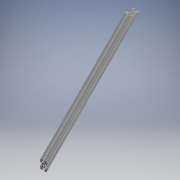
# Autodesk Inventor part: HFBL5-2020-300_
Saved by Autodesk Inventor 2017.3 (Build 213256000, 256)
## iProperties
Part Number: HFBL5-2020-300_
Material: Generic
Catalog Web Link: www.cadenas.de
Description: HFBL5_-Brackets HFS5 Frame Brackets for Reinforcement
Vendor: MISUMI
Document SubType Name: Modeling
Designer: partserver
Manufacturer: MISUMI
Mass: 73.1525 g
Surface Area: 703.124 cm^2
Volume: 73.1525 cm^3
Density: 1 g/cm^3
Appearance: PSOLRGB-192-192-192
Category: PARTsolutions
Company: MISUMI
Title: HFBL5-2020-300_
Author: Cadenas PARTsolutions
Comments: Brackets HFS5 Frame Brackets for Reinforcement
PSOL_IDENT_0: {$CADENAS_DATA\23d-libs\misumi\metric\38_al_extrusions_blackets\5\hfbl5.prj},176 {VTYP=3D},{NB=HFBL5
PSOL_IDENT_1: -2020-300_},{LINA=HFBL5-2020-300_},{NN=HFBL5_},{DATE=08.06.2021 08:25:15},{GEOMDATE=30.01.2015 00:00
PSOL_IDENT_2: :00},{VERSION=},{LINEID=10},{WBVAR=L,ALT},{WBNUMERIC=L}  {NB=HFBL5-2020-300_},{LINA=HFBL5-2020-300_}
PSOL_IDENT_3: ,{KT=1},{PN=HFBL5-2020-300},{TP=HFBL5},{NO=2020},{TYPE=HFBL5},{MAT=A6N01SS-T5},{ST=Alumite Treatment
PSOL_IDENT_4: (No surface treatment on the side cut at 45 degree and  Counterbore type)},{FEAT=4 Slots},{L=300},{
PSOL_IDENT_5: LTOL=+/- 0.5},{MASS=0.50},{SA=153},{GMILX=0.57x10^4},{GMILY=0.57x10^4},{WIDTH=20},{HEIGHT=20},{TAPDE
PSOL_IDENT_6: PTH=15},{TAPSTART=0},{DRILLLENGTH=0},{DRILLDIA=4.2},{TAPPOSHOR=0},{TAPPOSVER=0},{VER=1},{DIM=1},{CLF=
PSOL_IDENT_7: HFS5-2020},{ALT3=},{AB=CBM5-8},{ABQ=2},{AN=HNTT5-5},{ANQ=2},{ALT=}
NB: HFBL5-2020-300_
NN: HFBL5_
NT: Brackets HFS5 Frame Brackets for Reinforcement
NBSYN: $PN._
LINA: HFBL5-2020-300_
CATALOG: Misumi
PN: HFBL5-2020-300
NO: 2020
MAT: A6N01SS-T5 Aluminum Alloy
ST: Alumite Treatment (No surface treatment on the side cut at 45 degree and  Counterbore type)
L: 300
WIDTH: 20
AB: CBM5-8
ABQ: 2
AN: HNTT5-5
ANQ: 2
ALT: w/o Set of Applicable Bolt and Nut
SUPPLIER: MISUMI
ARTICLENO: HFBL5-2020-300_
BOMINFO: HFBL5-2020-300_
CREATOR: CADENAS GmbH
Autodesk Inventor part; units mm, degrees
sketch "Sketch_1" plane through (0, 0, 0) normal (0, -0.7071068, 0.7071068) x (1, 0, 0)
  arc A0 (-10, 205.432) -> (-9.7, 205.132) centre (-9.7, 205.432) ccw
  line L0 (-9.7, 205.132) -> (-8, 205.132)
  line L1 (-8, 205.132) -> (-8, 208.132)
  line L2 (-8, 208.132) -> (-7.0607, 208.132)
  line L3 (-7.0607, 208.132) -> (-4, 205.0714)
  line L4 (-4, 205.0714) -> (-4, 202.432)
  line L5 (-4, 202.432) -> (-3.7, 202.132)
  line L6 (-3.7, 202.132) -> (-4, 201.832)
  line L7 (-4, 201.832) -> (-4, 199.1927)
  line L8 (-4, 199.1927) -> (-7.0607, 196.132)
  line L9 (-7.0607, 196.132) -> (-8, 196.132)
  line L10 (-8, 196.132) -> (-8, 199.132)
  line L11 (-8, 199.132) -> (-9.7, 199.132)
  arc A1 (-9.7, 199.132) -> (-10, 198.832) centre (-9.7, 198.832) ccw
  line L12 (-10, 198.832) -> (-10, 193.132)
  arc A2 (-10, 193.132) -> (-9, 192.132) centre (-9, 193.132) ccw
  line L13 (-9, 192.132) -> (-3.3, 192.132)
  arc A3 (-3.3, 192.132) -> (-3, 192.432) centre (-3.3, 192.432) ccw
  line L14 (-3, 192.432) -> (-3, 194.132)
  line L15 (-3, 194.132) -> (-6, 194.132)
  line L16 (-6, 194.132) -> (-6, 195.0714)
  line L17 (-6, 195.0714) -> (-2.9393, 198.132)
  line L18 (-2.9393, 198.132) -> (-0.3, 198.132)
  line L19 (-0.3, 198.132) -> (0, 198.432)
  line L20 (0, 198.432) -> (0.3, 198.132)
  line L21 (0.3, 198.132) -> (2.9393, 198.132)
  line L22 (2.9393, 198.132) -> (6, 195.0714)
  line L23 (6, 195.0714) -> (6, 194.132)
  line L24 (6, 194.132) -> (3, 194.132)
  line L25 (3, 194.132) -> (3, 192.432)
  arc A4 (3, 192.432) -> (3.3, 192.132) centre (3.3, 192.432) ccw
  line L26 (3.3, 192.132) -> (9, 192.132)
  arc A5 (9, 192.132) -> (10, 193.132) centre (9, 193.132) ccw
  line L27 (10, 193.132) -> (10, 198.832)
  arc A6 (10, 198.832) -> (9.7, 199.132) centre (9.7, 198.832) ccw
  line L28 (9.7, 199.132) -> (8, 199.132)
  line L29 (8, 199.132) -> (8, 196.132)
  line L30 (8, 196.132) -> (7.0607, 196.132)
  line L31 (7.0607, 196.132) -> (4, 199.1927)
  line L32 (4, 199.1927) -> (4, 201.832)
  line L33 (4, 201.832) -> (3.7, 202.132)
  line L34 (3.7, 202.132) -> (4, 202.432)
  line L35 (4, 202.432) -> (4, 205.0714)
  line L36 (4, 205.0714) -> (7.0607, 208.132)
  line L37 (7.0607, 208.132) -> (8, 208.132)
  line L38 (8, 208.132) -> (8, 205.132)
  line L39 (8, 205.132) -> (9.7, 205.132)
  arc A7 (9.7, 205.132) -> (10, 205.432) centre (9.7, 205.432) ccw
  line L40 (10, 205.432) -> (10, 211.132)
  arc A8 (10, 211.132) -> (9, 212.132) centre (9, 211.132) ccw
  line L41 (9, 212.132) -> (3.3, 212.132)
  arc A9 (3.3, 212.132) -> (3, 211.832) centre (3.3, 211.832) ccw
  line L42 (3, 211.832) -> (3, 210.132)
  line L43 (3, 210.132) -> (6, 210.132)
  line L44 (6, 210.132) -> (6, 209.1927)
  line L45 (6, 209.1927) -> (2.9393, 206.132)
  line L46 (2.9393, 206.132) -> (0.3, 206.132)
  line L47 (0.3, 206.132) -> (0, 205.832)
  line L48 (0, 205.832) -> (-0.3, 206.132)
  line L49 (-0.3, 206.132) -> (-2.9393, 206.132)
  line L50 (-2.9393, 206.132) -> (-6, 209.1927)
  line L51 (-6, 209.1927) -> (-6, 210.132)
  line L52 (-6, 210.132) -> (-3, 210.132)
  line L53 (-3, 210.132) -> (-3, 211.832)
  arc A10 (-3, 211.832) -> (-3.3, 212.132) centre (-3.3, 211.832) ccw
  line L54 (-3.3, 212.132) -> (-9, 212.132)
  arc A11 (-9, 212.132) -> (-10, 211.132) centre (-9, 211.132) ccw
  line L55 (-10, 211.132) -> (-10, 205.432)
  circle A12 centre (0, 202.132) radius 2.1
  constraints: 112 end point, 24 point on circle, 13 centre point
extrude "Extrusion1" add sketch "Sketch_1" along normal mid plane 426.2641
sketch "Sketch_2" plane through (0, 0, 0) normal (0, 0, 1) x (1, 0, 0)
  line L0 (-50, -300) -> (50, -300)
  line L1 (50, -300) -> (50, 0)
  line L2 (50, 0) -> (-50, 0)
  line L3 (-50, 0) -> (-50, -300)
  constraints: 8 end point
extrude "Extrusion2" cut sketch "Sketch_2" along normal mid plane 1200
sketch "Sketch_3" plane through (0, 0, 0) normal (0, 1, 0) x (-1, 0, 0)
  line L0 (50, -300) -> (50, 0)
  line L1 (50, 0) -> (-50, 0)
  line L2 (-50, 0) -> (-50, -300)
  line L3 (-50, -300) -> (50, -300)
  constraints: 8 end point
extrude "Extrusion3" cut sketch "Sketch_3" along normal mid plane 1200
sketch "Sketch_4" plane through (0, 0, 0) normal (1, 0, 0) x (0, 1, 0)
  line L0 (0, 285.65) -> (30, 285.65)
  line L1 (30, 285.65) -> (30, 280.9)
  line L2 (30, 280.9) -> (3, 280.9)
  line L3 (3, 280.9) -> (3, 282.9)
  line L4 (3, 282.9) -> (0, 282.9)
  line L5 (0, 282.9) -> (0, 285.65)
  line L6 (0, 285.65) -> (30, 285.65)
  constraints: 14 end point
revolve "Revolution1" cut sketch "Sketch_4" angle 360 about axis through (0, 0, 285.65) along (0, -1, 0)
sketch "Sketch_5" plane through (0, 0, 0) normal (1, 0, 0) x (0, 1, 0)
  line L0 (285.65, 0) -> (285.65, 30)
  line L1 (285.65, 30) -> (290.4, 30)
  line L2 (290.4, 30) -> (290.4, 3)
  line L3 (290.4, 3) -> (288.4, 3)
  line L4 (288.4, 3) -> (288.4, 0)
  line L5 (288.4, 0) -> (285.65, 0)
  line L6 (285.65, 0) -> (285.65, 30)
  constraints: 14 end point
revolve "Revolution2" cut sketch "Sketch_5" angle 360 about axis through (0, 285.65, 0) along (0, 0, -1)
ref_plane "bolt1_XY" through (0, 3, 285.65) normal (0, 1, 0) x (1, 0, 0)
ref_plane "bolt1_YZ" through (0, 3, 285.65) normal (1, 0, 0) x (0, 0, -1)
ref_plane "bolt1_ZX" through (0, 3, 285.65) normal (0, 0, -1) x (0, 1, 0)
ref_plane "bolt2_XY" through (0, 285.65, 3) normal (0, 0, 1) x (1, 0, 0)
ref_plane "bolt2_YZ" through (0, 285.65, 3) normal (1, 0, 0) x (0, 1, 0)
ref_plane "bolt2_ZX" through (0, 285.65, 3) normal (0, 1, 0) x (0, 0, 1)
body "Solid1"
